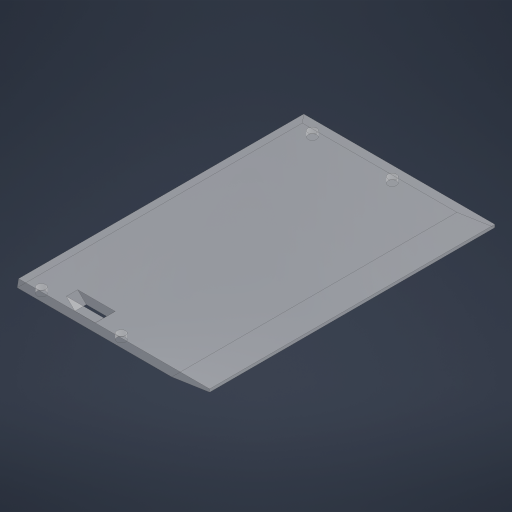
# Autodesk Inventor part: porywa
Saved by Autodesk Inventor 2024 (Build 280153000, 153)
## iProperties
Created: 2024-05-25
Part Number: porywa
Material: Polycarbonate, Clear
Document SubType Name: Modeling
Designer: Adam
Density: 1.2 g/cm^3
Appearance: Polycarbonate - Clear
Author: Adam
Autodesk Inventor part; units mm, degrees
ref_plane "YZ Plane" through (0, 0, 0) normal (1, 0, 0) x (0, 1, 0)
ref_plane "XZ Plane" through (0, 0, 0) normal (0, 1, 0) x (-1, 0, 0)
ref_plane "XY Plane" through (0, 0, 0) normal (0, 0, 1) x (1, 0, 0)
sketch "Sketch1" plane through (0, 0, 0) normal (0, 0, 1) x (1, 0, 0)
  line L0 (-24.865, 1.7403) -> (-25.3518, -1.2597)
  line L1 (-25.3518, -1.2597) -> (28.8493, -1.2597)
  line L2 (-24.865, 1.7403) -> (42.135, 1.7403)
  line L3 (42.135, 1.7403) -> (42.135, 0.7403)
  line L4 (42.135, 0.7403) -> (28.8493, -1.2597)
  point P0 (0, 0)
  dimension "d0" = 67
  dimension "d26" = 3
  dimension "d27" = 1
  dimension "d46" = 0.4868
  dimension "d48" = 13.2857
  constraints: 10 end point, 1 vertical
  measures "d0" distance of L0.start L2.end
  measures "d26" distance between parallel lines of L2 L1
  measures "d27" distance of L2.end L3.end
  measures "d46" horizontal distance of L0.end L0.start
  measures "d48" horizontal distance of L3.end L1.end
extrude "Extrusion1" add sketch "Sketch1" along normal blind 100
sketch "Sketch3" plane through (-24.865, 1.7403, 0) normal (0, 1, 0) x (1, 0, 0)
  line L0 (16.7348, -93) -> (23.8856, -93)
  line L1 (23.8856, -93) -> (23.8856, -97)
  line L2 (23.8856, -97) -> (16.7348, -97)
  line L3 (16.7348, -97) -> (16.7348, -93)
  point P0 (24.865, 0)
  point P1 (16.7856, -97)
  point P2 (23.8348, -93)
  constraints: 8 end point, 2 parallel, 1 horizontal, 1 perpendicular
extrude "Extrusion2" cut sketch "Sketch3" against normal through all
chamfer "Chamfer2" distance 3 angle 45 2 edges at (-8.1302, 1.7403, 95) (-0.9794, 1.7403, 95) measured on face at (-8.6302, 1.7403, 95) measured on face at (-0.4794, 1.7403, 95)
sketch "Sketch4" plane through (-25.3518, -1.2597, 0) normal (0, -1, 0) x (1, 0, 0)
  circle A0 centre (6, 97.5) radius 1.5
  circle A1 centre (34, 97.5) radius 1.5
  circle A2 centre (6, 2.5) radius 1.5
  circle A3 centre (34, 2.5) radius 1.5
  line L0 (0, 100) -> (54.2011, 100) projected
  line L1 (0, 0) -> (54.2011, 0) projected
  line L2 (0, 0) -> (0, 100) projected
  point P0 (25.3518, 0)
  dimension "d28" = 3
  dimension "d29" = 3
  dimension "d30" = 3
  dimension "d31" = 3
  dimension "d32" = 2.5
  dimension "d33" = 2.5
  dimension "d34" = 2.5
  dimension "d35" = 2.5
  dimension "d36" = 6
  dimension "d37" = 28
  dimension "d38" = 6
  dimension "d39" = 28
  constraints: 4 centre point
  measures "d28" diameter of A0
  measures "d29" diameter of A1
  measures "d30" diameter of A2
  measures "d31" diameter of A3
  measures "d32" distance from line of L0 A0.centre
  measures "d33" distance from line of L0 A1.centre
  measures "d34" distance from line of L1 A2.centre
  measures "d35" distance from line of L1 A3.centre
  measures "d36" distance from line of A0.centre L2
  measures "d37" distance of A1.centre A0.centre
  measures "d38" distance from line of L2 A2.centre
  measures "d39" distance of A3.centre A2.centre
extrude "Extrusion3" cut sketch "Sketch4" against normal blind 2
body "Solid1"
